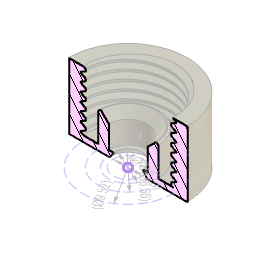
Magnetic PTFE Joiner (Insert) v11 (Autodesk Fusion 360 archive; units mm, degrees)
design "M10 Fitting"
Autodesk Fusion 360 part; units mm, degrees
sketch "M10 Housing" plane through (0, 0, 0) normal (0, 0, 1) x (1, 0, 0)
  circle A0 centre (0, 0) radius 4.76
  circle A1 centre (0, 0) radius 6.26
  dimension "d15" = 9.52
  dimension "d18" = 1.5
  constraint coincident A0.centre A1.centre
  measures "d15" diameter of A0
extrude "Extrude5" add sketch "M10 Housing" along normal blind 0.6 contours A0 | A1
extrude "Extrude6" add sketch "M10 Housing" along normal blind 6.3 from surface at 0.6
thread "Thread2" "ISO Metric profile 10.0 M10x0.9 6H" major diameter 10.1472 minor diameter 9.0355 pitch 0.9 angle 60 modelled right hand crest width 0.2248 on face at (4.7541, -0.2373, 4.8) crest through (4.5178, 0, 0.825)
sketch "Threading Seat" plane through (0, 0, 0.6) normal (0, 0, 1) x (1, 0, 0)
  circle A0 centre (0, 0) radius 3.2 construction
  circle A1 centre (0, 0) radius 3.18
  circle A2 centre (0, 0) radius 4.5178
  arc A3 (-3.1927, -3.1964) -> (3.1927, -3.1964) centre (0, 0) ccw
  spline S0 degree 3 poles (3.1927, -3.1964) (3.5831, -2.847) (3.9097, -2.4323) (4.4136, -1.5023) (4.5841, -0.9923) (4.7584, 0.1441) (4.7307, 0.7652) (4.4382, 1.9748) (4.1715, 2.5504) (3.4269, 3.5787) (2.9523, 4.0187) (1.8517, 4.7005) (1.2338, 4.9318) (0.5889, 5.0393) knots -1.080361 -1.080361 -1.080361 -1.080361 -0.922819 -0.922819 -0.762393 -0.762393 -0.577333 -0.577333 -0.38858 -0.38858 -0.196135 -0.196135 0 0 0 0
  arc A4 (0.5889, 5.0393) -> (-0.5889, 5.0393) centre (0, 0) ccw
  spline S1 degree 3 poles (-0.5889, 5.0393) (-1.1594, 4.9442) (-1.7094, 4.7521) (-2.7106, 4.1926) (-3.1558, 3.8323) (-3.944, 2.9276) (-4.2628, 2.3758) (-4.6648, 1.192) (-4.7486, 0.5731) (-4.6726, -0.6496) (-4.5183, -1.2418) (-3.9949, -2.3215) (-3.635, -2.8006) (-3.1927, -3.1964) knots -1.07772 -1.07772 -1.07772 -1.07772 -0.904601 -0.904601 -0.734359 -0.734359 -0.545242 -0.545242 -0.359808 -0.359808 -0.178061 -0.178061 0 0 0 0
  dimension "d32" = 6.4
  constraint coincident A0.centre A1.centre
  measures "d32" diameter of A0
extrude "Extrude7" add sketch "Threading Seat" along normal blind 3.2 contours A1
sketch "Catcher" plane through (0, 0, 3.8) normal (0, 0, 1) x (1, 0, 0)
  circle A0 centre (0, 0) radius 3.18
  circle A1 centre (0, 0) radius 2.05
  dimension "d37" = 4.1
  constraint coincident A0.centre A1.centre
  measures "d37" diameter of A1
extrude "Extrude8" cut sketch "Catcher" against normal up to surface (3.2 mm away) contours A1
sketch "PTFE Dimensions" plane through (0, 0, 0.6) normal (0, 0, 1) x (1, 0, 0)
  circle A0 centre (0, 0) radius 2.05
  circle A1 centre (0, 0) radius 1.55
  dimension "d40" = 3.1
  constraint coincident A0.centre A1.centre
  measures "d40" diameter of A1
extrude "Extrude9" cut sketch "PTFE Dimensions" against normal through all contours A1
chamfer "Chamfer1" distance 0.848 angle 45 1 edges at (-1.9113, 0.7413, 3.8)
chamfer "Chamfer4" distance 0.1878 angle 45 1 edges at (-2.9648, -1.1499, 3.8)
chamfer "Chamfer2" distance 0.42 distance2 0.6 1 edges at (-1.4451, -0.5605, 0) measured on face at (4.6609, 0.388, 0)
sketch "Summary Collection" plane through (0, 0, 0) normal (0, 0, 1) x (1, 0, 0)
  circle A0 centre (0, 0) radius 1.55 construction
  circle A1 centre (0, 0) radius 2.05 construction
  circle A2 centre (0, 0) radius 3.18 construction
  circle A3 centre (0, 0) radius 4.76 construction
  dimension "d47" = 3.1
  dimension "d48" = 4.1
  dimension "d49" = 6.36
  dimension "d50" = 9.52
  measures "d47" diameter of A0
  measures "d48" diameter of A1
  measures "d49" diameter of A2
  measures "d50" diameter of A3
sketch "Sketch7" plane through (0, 0, 0) normal (0, 0, 1) x (1, 0, 0)
  line L0 (-9.2466, 9.2174) -> (0, 9.2174)
  line L1 (0, 9.2174) -> (0, -9.2174)
  line L2 (0, -9.2174) -> (-9.2466, -9.2174)
  line L3 (-9.2466, -9.2174) -> (-9.2466, 9.2174)
  constraint horizontal L0
  constraint vertical L1
  constraint horizontal L2
  constraint vertical L3
  constraint midpoint L1 origin
extrude "Extrude10" [suppressed]
equation "WallThickness = 1.5 mm" comment "thickness of wall between M10 threading and edge of magnet"
equation "d18 = WallThickness"
equation "d27 = BottomThickness"
equation "d30 = ThreadingHeight"
equation "PrintTolerance = 0.02 mm"
equation "d34 = -PrintTolerance"
equation "d35 = InsertHeight"
equation "d38 = -BottomThickness"
equation "d43 = BottomThickness * 0.7"
equation "d44 = BottomThickness"
equation "BottomThickness = 0.6 mm"
equation "ThreadingHeight = 6.3 mm"
equation "InsertHeight = 3.2 mm"
